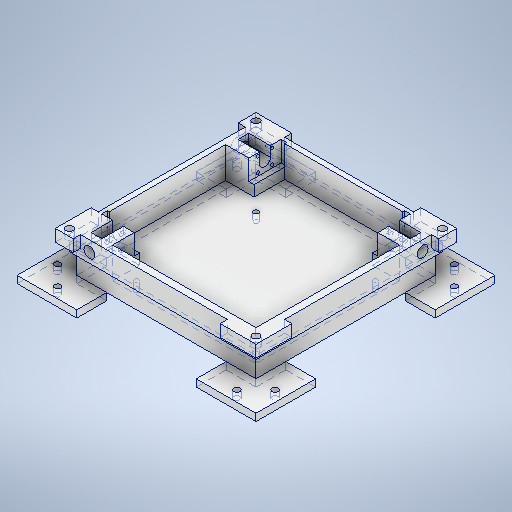
# Autodesk Inventor part: lower half
Saved by Autodesk Inventor 2025 (Build 290162000, 162)
## iProperties
Created: 2024-04-12
Part Number: lower half
Material: Aluminum 6061
Document SubType Name: Modeling
Designer: mahal
Density: 2.7 g/cm^3
Appearance: Aluminum - Flat
Mass: 892.67 g
Surface Area: 1106.39 cm^2
Volume: 330.618 cm^3
Author: mahal
Autodesk Inventor part; units mm, degrees
sketch "Sketch1" plane through (0, 0, 0) normal (0, 1, 0) x (-1, 0, 0)
  line L0 (75, 75) -> (-75, 75)
  line L1 (-75, 75) -> (-75, -75)
  line L2 (-75, -75) -> (75, -75)
  line L3 (75, -75) -> (75, 75)
  line L4 (75, 75) -> (-75, -75) construction
  line L5 (-75, 75) -> (75, -75) construction
  point P0 (0, 0)
  dimension "d0" = 150
  dimension "d1" = 150
  constraints: 12 end point, 2 midpoint, 2 parallel, 1 horizontal, 1 perpendicular
  measures "d0" distance of L2.end L1.end
  measures "d1" distance of L1.end L0.end
extrude "Extrusion1" add sketch "Sketch1" along normal blind 30
ref_plane "Work Plane1" through (0, 30, 0) normal (0, 1, 0) x (1, 0, 0)
sketch "Sketch2" plane through (0, 30, 0) normal (0, 1, 0) x (1, 0, 0)
  line L0 (72, -72) -> (-72, -72)
  line L1 (-72, -72) -> (-72, 72)
  line L2 (-72, 72) -> (72, 72)
  line L3 (72, 72) -> (72, -72)
  line L4 (72, -72) -> (-72, 72) construction
  line L5 (-72, -72) -> (72, 72) construction
  line L6 (72, -72) -> (-48, -72)
  line L7 (-48, -72) -> (-48, 48)
  line L8 (-48, 48) -> (72, 48)
  line L9 (72, 48) -> (72, -72)
  point P0 (0, 0)
  dimension "d5" = 144
  dimension "d6" = 144
  dimension "d7" = 120
  dimension "d8" = 120
  constraints: 20 end point, 4 parallel, 2 horizontal, 2 midpoint, 2 perpendicular
  measures "d5" distance of L1.end L2.end
  measures "d6" distance of L0.end L1.end
  measures "d7" distance of L7.end L8.end
  measures "d8" distance of L6.end L7.end
extrude "Extrusion2" cut sketch "Sketch2" against normal blind 26 contours L0 L7 L8 L3
sketch "Sketch3" plane through (0, 30, 0) normal (0, 1, 0) x (1, 0, 0)
  line L0 (72, -72) -> (-48, -72) projected
  line L1 (-48, -72) -> (-75, -72)
  line L2 (-75, 75) -> (-75, -75) projected
  line L3 (-61.5, -72) -> (-66, -72)
  line L4 (-61.5, -72) -> (-57, -72)
  line L5 (-57, -72) -> (-57, -54)
  line L6 (-57, -54) -> (-66, -54)
  line L7 (-66, -54) -> (-66, -72)
  line L8 (-57, -54) -> (-48, -54)
  line L9 (-48, -54) -> (-48, -49.5)
  line L10 (-48, -49.5) -> (-75, -49.5)
  line L11 (-75, -54) -> (-66, -54)
  line L12 (-75, -54) -> (-75, -49.5)
  line L13 (-48, 48) -> (72, 48) projected
  line L14 (72, 48) -> (72, 75)
  line L15 (72, 61.5) -> (72, 57)
  line L16 (72, 61.5) -> (72, 66)
  line L17 (72, 66) -> (54, 66)
  line L18 (54, 66) -> (54, 57)
  line L19 (54, 57) -> (72, 57)
  line L20 (54, 57) -> (54, 48)
  line L21 (54, 48) -> (49.5, 48)
  line L22 (49.5, 48) -> (49.5, 75)
  line L23 (75, 75) -> (-75, 75) projected
  line L24 (49.5, 75) -> (54, 75)
  line L25 (54, 75) -> (54, 66)
  line L26 (0, 48) -> (0, 57)
  line L27 (48, 48) -> (-72, 48)
  line L28 (-72, 48) -> (-72, 75)
  line L29 (-72, 61.5) -> (-72, 57)
  line L30 (-72, 61.5) -> (-72, 66)
  line L31 (-72, 66) -> (-54, 66)
  line L32 (-54, 66) -> (-54, 57)
  line L33 (-54, 57) -> (-72, 57)
  line L34 (-54, 57) -> (-54, 48)
  line L35 (-54, 48) -> (-49.5, 48)
  line L36 (-49.5, 48) -> (-49.5, 75)
  line L37 (-75, 75) -> (75, 75)
  line L38 (-49.5, 75) -> (-54, 75)
  line L39 (-54, 75) -> (-54, 66)
  point P0 (0, 0)
  dimension "d11" = 4.5
  dimension "d12" = 4.5
  dimension "d13" = 18
  dimension "d14" = 4.5
  dimension "d15" = 4.5
  dimension "d16" = 4.5
  dimension "d17" = 18
  dimension "d18" = 4.5
  constraints: 72 end point, 19 point on line, 14 symmetric about line, 12 perpendicular, 3 vertical, 2 horizontal, 2 midpoint, 1 collinear
  measures "d11" distance of L3.start L3.end
  measures "d12" distance of L3.start L4.end
  measures "d13" distance of L4.end L5.end
  measures "d14" distance of L8.end L9.end
  measures "d15" distance of L15.start L15.end
  measures "d16" distance of L15.start L16.end
  measures "d17" distance of L16.end L17.end
  measures "d18" distance of L20.end L21.end
extrude "Extrusion3" cut sketch "Sketch3" against normal blind 12.5 contours L1 L7 L6 L5 | L6 L11 L2 L10 L9 L8 | L23 L36 L27 L34 L32 L39 | L31 L32 L33 L28 | L23 L25 L18 L20 L13 L22 | L17 L14 L19 L18
sketch "Sketch5" plane through (0, 30, 0) normal (0, 1, 0) x (1, 0, 0)
  line L0 (54, 57) -> (54, 48) projected
  line L1 (49.5, 48) -> (49.5, 75) projected
  line L2 (54, 48) -> (49.5, 48)
  line L3 (49.5, 48) -> (49.5, 75)
  line L4 (49.5, 75) -> (54, 75)
  line L5 (54, 75) -> (54, 48)
  line L6 (-49.5, 75) -> (-49.5, 48) projected
  line L7 (-54, 66) -> (-54, 75) projected
  line L8 (-49.5, 48) -> (-54, 48)
  line L9 (-54, 48) -> (-54, 75)
  line L10 (-54, 75) -> (-49.5, 75)
  line L11 (-49.5, 75) -> (-49.5, 48)
  line L12 (-75, -49.5) -> (-48, -49.5) projected
  line L13 (-48, -54) -> (-75, -54)
  line L14 (-75, -54) -> (-75, -49.5)
  line L15 (-75, -49.5) -> (-48, -49.5)
  line L16 (-48, -49.5) -> (-48, -54)
  point P0 (0, 0)
  constraints: 24 end point, 6 parallel, 3 horizontal, 3 perpendicular
extrude "Extrusion4" cut sketch "Sketch5" against normal blind 17
sketch "Sketch6" plane through (0, 30, 0) normal (0, 1, 0) x (1, 0, 0)
  line L0 (49.5, 48) -> (49.5, 75) projected
  line L1 (49.5, 48) -> (-48.9491, 48)
  line L2 (-48.9491, 48) -> (-48.9491, 73.5)
  line L3 (-48.9491, 73.5) -> (49.5, 73.5)
  line L4 (49.5, 73.5) -> (49.5, 48)
  line L5 (-48, -49.5) -> (-48, 48) projected
  line L6 (-75, 75) -> (-75, -49.5) projected
  line L7 (-48, -49.5) -> (-75, -49.5)
  line L8 (-75, -49.5) -> (-75, 48)
  line L9 (-75, 48) -> (-48, 48)
  line L10 (-48, 48) -> (-48, -49.5)
  line L11 (-48, -49.5) -> (-73.5, -49.5)
  line L12 (-73.5, -49.5) -> (-73.5, 48)
  line L13 (-73.5, 48) -> (-48, 48)
  line L14 (-48, 48) -> (-48, -49.5)
  point P0 (0, 0)
  dimension "d23" = 25.5
  dimension "d24" = 25.5
  constraints: 24 end point, 6 parallel, 3 horizontal, 3 perpendicular, 3 point on line
  measures "d23" distance of L1.end L2.end
  measures "d24" distance of L12.end L13.end
extrude "Extrusion5" cut sketch "Sketch6" against normal up to surface (26 mm away) contours L1 L2 L3 L0 | L5 L7 L12 L9 L1
sketch "Sketch7" plane through (0, 30, 0) normal (0, 1, 0) x (1, 0, 0)
  line L0 (78, -78) -> (-78, -78)
  line L1 (-78, -78) -> (-78, 78)
  line L2 (-78, 78) -> (78, 78)
  line L3 (78, 78) -> (78, -78)
  line L4 (78, -78) -> (-78, 78) construction
  line L5 (-78, -78) -> (78, 78) construction
  line L6 (-75, 75) -> (-75, -49.5) projected
  line L7 (75, -75) -> (-75, -75)
  line L8 (-75, -75) -> (-75, 75)
  line L9 (-75, 75) -> (75, 75)
  line L10 (75, 75) -> (75, -75)
  line L11 (75, -75) -> (-75, 75) construction
  line L12 (-75, -75) -> (75, 75) construction
  point P0 (0, 0)
  dimension "d27" = 156
  dimension "d28" = 156
  constraints: 24 end point, 4 midpoint, 4 parallel, 2 horizontal, 2 perpendicular
  measures "d27" distance of L1.end L2.end
  measures "d28" distance of L0.end L1.end
extrude "Extrusion6" add sketch "Sketch7" against normal up to surface (17 mm away)
ref_plane "Work Plane2" through (-48.9491, 4, -73.5) normal (1, 0, 0) x (0, 0, -1)
sketch "Sketch8" plane through (-48.9491, 4, -73.5) normal (1, 0, 0) x (0, 0, -1)
  line L0 (-25.5, 26) -> (0, 26) projected
  line L1 (-25.5, 26) -> (0, 26)
  line L2 (0, 26) -> (0, 0)
  line L3 (0, 0) -> (-25.5, 0)
  line L4 (-25.5, 0) -> (-25.5, 26)
  point P0 (-73.5, -4)
  constraints: 8 end point, 2 parallel, 1 horizontal, 1 perpendicular
extrude "Extrusion7" cut sketch "Sketch8" against normal up to surface (0.5509 mm away)
sketch "Sketch9" plane through (0, 30, 0) normal (0, 1, 0) x (1, 0, 0)
  line L0 (-78, -78) -> (78, -78) projected
  line L1 (-78, -78) -> (-78, -54)
  line L2 (-78, 78) -> (-78, -78) projected
  line L3 (-78, -54) -> (-84, -54)
  line L4 (-84, -54) -> (-84, -78)
  line L5 (-84, -78) -> (-84, -84)
  line L6 (-84, -84) -> (-78, -84)
  line L7 (-78, -84) -> (-54, -84)
  line L8 (-54, -84) -> (-54, -78)
  line L9 (-78, -78) -> (-54, -78)
  line L10 (-78, 0) -> (-59.442, 0)
  line L11 (0, -78) -> (0, -66)
  line L12 (72, -72) -> (-48, -72) projected
  line L13 (-78, 78) -> (-78, 54)
  line L14 (-78, 54) -> (-84, 54)
  line L15 (-84, 54) -> (-84, 78)
  line L16 (-84, 78) -> (-84, 84)
  line L17 (-84, 84) -> (-78, 84)
  line L18 (-78, 84) -> (-54, 84)
  line L19 (-54, 84) -> (-54, 78)
  line L20 (-78, 78) -> (-54, 78)
  line L21 (78, -78) -> (-78, -78)
  line L22 (78, -78) -> (78, -54)
  line L23 (78, -54) -> (84, -54)
  line L24 (84, -54) -> (84, -78)
  line L25 (84, -78) -> (84, -84)
  line L26 (84, -84) -> (78, -84)
  line L27 (78, -84) -> (54, -84)
  line L28 (54, -84) -> (54, -78)
  line L29 (78, 78) -> (78, -78)
  line L30 (78, 78) -> (78, 54)
  line L31 (78, 54) -> (84, 54)
  line L32 (84, 54) -> (84, 78)
  line L33 (84, 78) -> (84, 84)
  line L34 (78, 84) -> (54, 84)
  line L35 (84, 84) -> (78, 84)
  line L36 (54, 84) -> (54, 78)
  line L37 (78, 78) -> (54, 78)
  point P0 (0, 0)
  dimension "d34" = 24
  dimension "d35" = 6
  dimension "d36" = 6
  dimension "d37" = 24
  constraints: 70 end point, 25 symmetric about line, 11 point on line, 4 perpendicular, 2 horizontal, 2 midpoint, 1 collinear
  measures "d34" distance of L0.start L1.end
  measures "d35" distance of L1.end L3.end
  measures "d36" distance of L4.end L5.end
  measures "d37" distance of L6.end L7.end
extrude "Extrusion8" add sketch "Sketch9" against normal blind 10
sketch "Sketch10" plane through (0, 30, 0) normal (0, 1, 0) x (1, 0, 0)
  line L0 (-84, 54) -> (-84, 84) projected
  line L1 (-78, 54) -> (-78, 78) projected
  line L2 (-84, 84) -> (-78, 84)
  line L3 (-78, 84) -> (-78, 78)
  line L4 (-78, 78) -> (-84, 78)
  line L5 (-84, 78) -> (-84, 84)
  circle A0 centre (-78, 78) radius 3
  line L6 (78, 78) -> (-78, 78) projected
  line L7 (0, 78) -> (0, 61.3441)
  line L8 (-78, 54) -> (-78, -54) projected
  line L9 (-78, 0) -> (-60.0355, 0)
  circle A1 centre (78, 78) radius 3
  circle A2 centre (-78, -78) radius 3
  circle A3 centre (78, -78) radius 3
  point P0 (0, 0)
  dimension "d40" = 6
  constraints: 12 end point, 4 centre point, 3 symmetric about line, 2 horizontal, 2 midpoint, 2 parallel, 1 coincident, 1 perpendicular, 1 vertical, 3 other
  measures "d40" diameter of A0
extrude "Extrusion9" cut sketch "Sketch10" against normal blind 7 contours A1 | A0 L3 L4 | L4 L1 A0 | L6 A0 L1 | L3 A0 L6 | A2 | A3
ref_plane "Work Plane3" through (0, 4, 0) normal (0, 1, 0) x (1, 0, 0)
sketch "Sketch11" plane through (0, 4, 0) normal (0, 1, 0) x (1, 0, 0)
  line L0 (72, -72) -> (-48, -72) projected
  line L1 (72, -72) -> (62, -72)
  line L2 (62, -72) -> (62, -62)
  line L3 (62, -62) -> (72, -62)
  line L4 (72, -62) -> (72, -72)
  circle A0 centre (62, -62) radius 2
  line L5 (72, -72) -> (-48, -72)
  line L6 (-48, -72) -> (-48, 48)
  line L7 (-48, 48) -> (72, 48)
  line L8 (72, 48) -> (72, -72)
  line L9 (12, -72) -> (12, -54.0613)
  line L10 (12, -12) -> (26.1191, -12)
  circle A1 centre (-38, -62) radius 2
  circle A2 centre (62, 38) radius 2
  circle A3 centre (-38, 38) radius 2
  point P0 (0, 0)
  dimension "d44" = 10
  dimension "d45" = 10
  dimension "d46" = 4
  dimension "d47" = 120
  dimension "d48" = 120
  constraints: 20 end point, 4 centre point, 4 parallel, 3 horizontal, 3 symmetric about line, 2 perpendicular, 1 coincident, 1 midpoint, 1 vertical, 3 other
  measures "d44" distance of L2.end L3.end
  measures "d45" distance of L1.end L2.end
  measures "d46" diameter of A0
  measures "d47" distance of L6.end L7.end
  measures "d48" distance of L5.end L6.end
extrude "Extrusion10" cut sketch "Sketch11" against normal blind 8 contours A0 L3 L2 | L2 L3 A0 | A1 | A2 | A3
ref_plane "Work Plane4" through (0, 0, 0) normal (0, -1, 0) x (1, 0, 0)
sketch "Sketch12" plane through (0, 0, 0) normal (0, -1, 0) x (1, 0, 0)
  line L0 (-75, 75) -> (75, 75) projected
  line L1 (-75, 75) -> (75, 75)
  line L2 (75, 75) -> (75, -75)
  line L3 (75, -75) -> (-75, -75)
  line L4 (-75, -75) -> (-75, 75)
  point P0 (0, 0)
  constraints: 8 end point, 2 parallel, 1 horizontal, 1 perpendicular
extrude "Extrusion11" add sketch "Sketch12" along normal blind 4
ref_plane "Work Plane5" through (0, -4, 0) normal (0, -1, 0) x (1, 0, 0)
sketch "Sketch13" plane through (0, -4, 0) normal (0, -1, 0) x (1, 0, 0)
  line L0 (-100, -100) -> (100, -100)
  line L1 (100, -100) -> (100, 100)
  line L2 (100, 100) -> (-100, 100)
  line L3 (-100, 100) -> (-100, -100)
  line L4 (-100, -100) -> (100, 100) construction
  line L5 (100, -100) -> (-100, 100) construction
  line L6 (75, -75) -> (75, 75) projected
  line L7 (-75, -75) -> (75, -75)
  line L8 (75, -75) -> (75, 75)
  line L9 (75, 75) -> (-75, 75)
  line L10 (-75, 75) -> (-75, -75)
  line L11 (-75, -75) -> (75, 75) construction
  line L12 (75, -75) -> (-75, 75) construction
  line L13 (-100, -100) -> (-50, -100)
  line L14 (-50, -100) -> (-50, -50)
  line L15 (-50, -50) -> (-100, -50)
  line L16 (-100, -50) -> (-100, -100)
  line L17 (-100, -100) -> (-50, -50) construction
  line L18 (-50, -100) -> (-100, -50) construction
  line L19 (-100, 50) -> (-50, 50)
  line L20 (-50, 50) -> (-50, 100)
  line L21 (-50, 100) -> (-100, 100)
  line L22 (-100, 100) -> (-100, 50)
  line L23 (-100, 50) -> (-50, 100) construction
  line L24 (-50, 50) -> (-100, 100) construction
  line L25 (50, 50) -> (100, 50)
  line L26 (100, 50) -> (100, 100)
  line L27 (100, 100) -> (50, 100)
  line L28 (50, 100) -> (50, 50)
  line L29 (50, 50) -> (100, 100) construction
  line L30 (100, 50) -> (50, 100) construction
  line L31 (50, -100) -> (100, -100)
  line L32 (100, -100) -> (100, -50)
  line L33 (100, -50) -> (50, -50)
  line L34 (50, -50) -> (50, -100)
  line L35 (50, -100) -> (100, -50) construction
  line L36 (100, -100) -> (50, -50) construction
  point P0 (0, 0)
  point P1 (50, -75)
  point P2 (75, -50)
  point P3 (50, 75)
  point P4 (75, 50)
  point P5 (-50, 75)
  point P6 (-75, 50)
  point P7 (-75, -50)
  point P8 (-50, -75)
  dimension "d55" = 200
  dimension "d56" = 200
  dimension "d57" = 50
  dimension "d58" = 50
  dimension "d59" = 50
  dimension "d60" = 50
  dimension "d61" = 50
  dimension "d62" = 50
  dimension "d63" = 50
  constraints: 72 end point, 12 midpoint, 12 parallel, 6 horizontal, 6 perpendicular, 1 point on line
  measures "d55" distance of L2.end L1.end
  measures "d56" distance of L1.end L0.end
  measures "d57" distance of L15.end L14.end
  measures "d58" distance of L21.end L20.end
  measures "d59" distance of L20.end L19.end
  measures "d60" distance of L27.end L1.end
  measures "d61" distance of L1.end L25.end
  measures "d62" distance of L33.end L32.end
  measures "d63" distance of L32.end L31.end
extrude "Extrusion12" add sketch "Sketch13" along normal blind 6 contours L3 L15 L10 L7 L14 L0 | L34 L7 L6 L33 L1 L0 | L3 L2 L20 L9 L10 L19 | L25 L6 L9 L28 L2 L1
ref_plane "Work Plane6" through (0, -4, 0) normal (0, 1, 0) x (1, 0, 0)
sketch "Sketch14" plane through (0, -4, 0) normal (0, 1, 0) x (1, 0, 0)
  line L0 (100, -50) -> (100, -100) projected
  line L1 (100, -100) -> (100, -50)
  line L2 (50, -100) -> (50, -75) projected
  line L3 (100, -100) -> (50, -100)
  line L4 (75, -100) -> (75, -91)
  line L5 (100, -75) -> (91, -75)
  circle A0 centre (91, -75) radius 2.5
  circle A1 centre (75, -91) radius 2.5
  line L6 (-78, -78) -> (78, -78) projected
  line L7 (0, -78) -> (0, -91)
  line L8 (78, 0) -> (95.5, 0)
  circle A2 centre (-91, -75) radius 2.5
  circle A3 centre (-75, -91) radius 2.5
  circle A4 centre (91, 75) radius 2.5
  circle A5 centre (75, 91) radius 2.5
  circle A6 centre (-75, 91) radius 2.5
  circle A7 centre (-91, 75) radius 2.5
  point P0 (0, 0)
  dimension "d67" = 9
  dimension "d68" = 9
  dimension "d69" = 5
  dimension "d70" = 5
  constraints: 12 end point, 8 centre point, 6 symmetric about line, 3 midpoint, 2 coincident, 2 horizontal, 2 vertical, 1 collinear, 1 perpendicular, 6 other
  measures "d67" distance of L4.start L4.end
  measures "d68" distance of L5.start L5.end
  measures "d69" diameter of A0
  measures "d70" diameter of A1
extrude "Extrusion13" cut sketch "Sketch14" against normal up to surface (6 mm away)
ref_plane "Work Plane7" through (72, 17.5, -66) normal (-1, 0, 0) x (0, 0, 1)
sketch "Sketch15" plane through (72, 17.5, -66) normal (-1, 0, 0) x (0, 0, 1)
  line L0 (0, 12.5) -> (9, 12.5) projected
  line L1 (4.5, 12.5) -> (4.5, 4)
  circle A0 centre (4.5, 4) radius 4.5
  point P0 (66, -17.5)
  dimension "d74" = 8.5
  dimension "d75" = 9
  constraints: 2 end point, 1 centre point, 1 coincident, 1 midpoint, 1 vertical
  measures "d74" distance of L1.start L1.end
  measures "d75" diameter of A0
extrude "Extrusion14" cut sketch "Sketch15" against normal up to surface (12 mm away)
ref_plane "Work Plane8" through (-72, 17.5, -57) normal (1, 0, 0) x (0, 0, -1)
sketch "Sketch16" plane through (-72, 17.5, -57) normal (1, 0, 0) x (0, 0, -1)
  line L0 (0, 12.5) -> (9, 12.5) projected
  line L1 (4.5, 12.5) -> (4.5, 4)
  circle A0 centre (4.5, 4) radius 4.5
  point P0 (-57, -17.5)
  dimension "d79" = 8.5
  dimension "d80" = 9
  constraints: 2 end point, 1 centre point, 1 coincident, 1 midpoint, 1 vertical
  measures "d79" distance of L1.start L1.end
  measures "d80" diameter of A0
extrude "Extrusion15" cut sketch "Sketch16" against normal up to surface (12 mm away)
ref_plane "Work Plane9" through (-57, 30, 72) normal (0, 0, -1) x (-1, 0, 0)
sketch "Sketch17" plane through (-57, 30, 72) normal (0, 0, -1) x (-1, 0, 0)
  line L0 (0, 0) -> (9, 0) projected
  line L1 (4.5, 0) -> (4.5, -9)
  circle A0 centre (4.5, -9) radius 4.5
  point P0 (-57, -30)
  dimension "d84" = 9
  dimension "d85" = 9
  constraints: 2 end point, 1 centre point, 1 coincident, 1 midpoint, 1 vertical
  measures "d84" distance of L1.start L1.end
  measures "d85" diameter of A0
extrude "Extrusion16" cut sketch "Sketch17" against normal up to surface (12 mm away)
ref_plane "Work Plane10" through (0, 30, 0) normal (0, 1, 0) x (1, 0, 0)
sketch "Sketch18" plane through (0, 30, 0) normal (0, 1, 0) x (1, 0, 0)
  line L0 (78, -54) -> (78, 54) projected
  line L1 (84, 54) -> (84, 84) projected
  line L2 (78, 54) -> (84, 54)
  line L3 (84, 54) -> (84, 69)
  line L4 (84, 69) -> (78, 69)
  line L5 (78, 69) -> (78, 54)
  line L6 (-84, 84) -> (-84, 54) projected
  line L7 (-78, 54) -> (-84, 54)
  line L8 (-84, 54) -> (-84, 69)
  line L9 (-84, 69) -> (-78, 69)
  line L10 (-78, 69) -> (-78, 54)
  line L11 (-54, -78) -> (-54, -84) projected
  line L12 (-65.8875, -84) -> (-84, -84) projected
  line L13 (-54, -78) -> (-69, -78)
  line L14 (-69, -78) -> (-69, -84)
  line L15 (-69, -84) -> (-54, -84)
  line L16 (-54, -84) -> (-54, -78)
  point P0 (0, 0)
  dimension "d89" = 15
  constraints: 24 end point, 6 parallel, 3 horizontal, 3 perpendicular, 2 midpoint, 2 point on line
  measures "d89" distance of L15.end L14.end
extrude "Extrusion17" cut sketch "Sketch18" against normal up to surface (10 mm away)
sketch "Sketch19" plane through (72, 17.5, -66) normal (-1, 0, 0) x (0, 0, 1)
  arc A0 (9, 4) -> (0, 4) centre (4.5, 4) ccw projected
  circle A1 centre (4.5, 4) radius 4.5
  line L0 (0, 4) -> (9, 4)
  line L1 (9, 4) -> (9, -0.5)
  line L2 (9, -0.5) -> (0, -0.5)
  line L3 (0, -0.5) -> (0, 4)
  point P0 (66, -17.5)
  point P1 (4.5, -0.5)
  constraints: 8 end point, 2 parallel, 1 centre point, 1 coincident, 1 horizontal, 1 perpendicular
extrude "Extrusion18" add sketch "Sketch19" along normal up to surface (18 mm away) contours L1 L2 A1 | A1 L2 L3
sketch "Sketch20" plane through (72, 17.5, -66) normal (-1, 0, 0) x (0, 0, 1)
  arc A0 (9, 4) -> (0, 4) centre (4.5, 4) ccw projected
  circle A1 centre (4.5, 4) radius 4.5
  point P0 (66, -17.5)
  constraints: 1 centre point, 1 coincident
extrude "Extrusion19" cut sketch "Sketch20" along normal up to surface (18 mm away)
sketch "Sketch21" plane through (-72, 17.5, -57) normal (1, 0, 0) x (0, 0, -1)
  arc A0 (9, 4) -> (0, 4) centre (4.5, 4) ccw projected
  circle A1 centre (4.5, 4) radius 4.5
  line L0 (0, 4) -> (9, 4)
  line L1 (9, 4) -> (9, -0.5)
  line L2 (9, -0.5) -> (0, -0.5)
  line L3 (0, -0.5) -> (0, 4)
  point P0 (-57, -17.5)
  point P1 (4.5, -0.5)
  constraints: 8 end point, 2 parallel, 1 centre point, 1 coincident, 1 horizontal, 1 perpendicular
extrude "Extrusion20" add sketch "Sketch21" along normal up to surface (18 mm away) contours L1 L2 A1 | A1 L2 L3
sketch "Sketch22" plane through (-72, 17.5, -57) normal (1, 0, 0) x (0, 0, -1)
  arc A0 (9, 4) -> (0, 4) centre (4.5, 4) ccw projected
  circle A1 centre (4.5, 4) radius 4.5
  point P0 (-57, -17.5)
  constraints: 1 centre point, 1 coincident
extrude "Extrusion21" cut sketch "Sketch22" along normal up to surface (18 mm away)
sketch "Sketch23" plane through (-57, 30, 72) normal (0, 0, -1) x (-1, 0, 0)
  arc A0 (9, -9) -> (0, -9) centre (4.5, -9) ccw projected
  circle A1 centre (4.5, -9) radius 4.5
  line L0 (9, -9) -> (0, -9)
  line L1 (0, -9) -> (0, -13.5)
  line L2 (0, -13.5) -> (9, -13.5)
  line L3 (9, -13.5) -> (9, -9)
  point P0 (-57, -30)
  point P1 (4.5, -13.5)
  constraints: 8 end point, 2 parallel, 1 centre point, 1 coincident, 1 horizontal, 1 perpendicular
extrude "Extrusion22" add sketch "Sketch23" along normal up to surface (18 mm away) contours L3 L2 A1 | A1 L2 L1
sketch "Sketch24" plane through (-57, 30, 72) normal (0, 0, -1) x (-1, 0, 0)
  arc A0 (9, -9) -> (0, -9) centre (4.5, -9) ccw projected
  circle A1 centre (4.5, -9) radius 4.5
  point P0 (-57, -30)
  constraints: 1 centre point, 1 coincident
extrude "Extrusion23" cut sketch "Sketch24" along normal up to surface (18 mm away)
ref_plane "Work Plane11" through (54, 30, -57) normal (-1, 0, 0) x (0, 0, 1)
sketch "Sketch25" plane through (54, 30, -57) normal (-1, 0, 0) x (0, 0, 1)
  line L0 (-18, -17) -> (-18, 0) projected
  line L1 (-18, 0) -> (9, 0)
  line L2 (9, 0) -> (9, -17)
  line L3 (9, -17) -> (-18, -17)
  line L4 (-18, -17) -> (-18, 0)
  line L5 (-13, 0) -> (4, 0)
  line L6 (4, 0) -> (4, -17)
  line L7 (4, -17) -> (-13, -17)
  line L8 (-13, -17) -> (-13, 0)
  arc A0 (-9, -8.5) -> (0, -8.5) centre (-4.5, -8.5) ccw projected
  line L9 (-13, 0) -> (4, -17) construction
  line L10 (4, 0) -> (-13, -17) construction
  line L11 (-10.5, -2.5) -> (1.5, -2.5)
  line L12 (1.5, -2.5) -> (1.5, -14.5)
  line L13 (1.5, -14.5) -> (-10.5, -14.5)
  line L14 (-10.5, -14.5) -> (-10.5, -2.5)
  line L15 (-10.5, -2.5) -> (1.5, -14.5) construction
  line L16 (1.5, -2.5) -> (-10.5, -14.5) construction
  circle A1 centre (-10.5, -2.5) radius 1.25
  circle A2 centre (1.5, -2.5) radius 1.25
  circle A3 centre (1.5, -14.5) radius 1.25
  circle A4 centre (-10.5, -14.5) radius 1.25
  point P0 (57, -30)
  dimension "d105" = 17
  dimension "d106" = 12
  dimension "d107" = 12
  dimension "d108" = 2.5
  dimension "d109" = 2.5
  dimension "d110" = 2.5
  dimension "d111" = 2.5
  constraints: 32 end point, 6 parallel, 4 centre point, 4 coincident, 4 midpoint, 3 horizontal, 3 perpendicular, 1 point on line
  measures "d105" distance of L6.end L7.end
  measures "d106" distance of L12.end L13.end
  measures "d107" distance of L11.end L12.end
  measures "d108" diameter of A1
  measures "d109" diameter of A2
  measures "d110" diameter of A3
  measures "d111" diameter of A4
extrude "Extrusion24" cut sketch "Sketch25" against normal blind 4 contours L14 A1 L11 | L11 A1 L14 | A2 L12 L11 | L11 L12 A2 | A4 L13 L14 | L14 L13 A4 | A3 L13 L12 | L12 L13 A3
ref_plane "Work Plane12" through (-54, 13, -48) normal (1, 0, 0) x (0, 0, -1)
sketch "Sketch26" plane through (-54, 13, -48) normal (1, 0, 0) x (0, 0, -1)
  line L0 (5, 17) -> (22, 17)
  line L1 (22, 17) -> (22, 0)
  line L2 (22, 0) -> (5, 0)
  line L3 (5, 0) -> (5, 17)
  arc A0 (9, 8.5) -> (18, 8.5) centre (13.5, 8.5) ccw projected
  line L4 (5, 17) -> (22, 0) construction
  line L5 (22, 17) -> (5, 0) construction
  line L6 (7.5, 14.5) -> (19.5, 14.5)
  line L7 (19.5, 14.5) -> (19.5, 2.5)
  line L8 (19.5, 2.5) -> (7.5, 2.5)
  line L9 (7.5, 2.5) -> (7.5, 14.5)
  line L10 (7.5, 14.5) -> (19.5, 2.5) construction
  line L11 (19.5, 14.5) -> (7.5, 2.5) construction
  circle A1 centre (7.5, 14.5) radius 1.25
  circle A2 centre (19.5, 14.5) radius 1.25
  circle A3 centre (19.5, 2.5) radius 1.25
  circle A4 centre (7.5, 2.5) radius 1.25
  point P0 (-48, -13)
  dimension "d115" = 17
  dimension "d116" = 17
  dimension "d117" = 12
  dimension "d118" = 12
  dimension "d119" = 2.5
  dimension "d120" = 2.5
  dimension "d121" = 2.5
  dimension "d122" = 2.5
  constraints: 24 end point, 5 midpoint, 4 centre point, 4 coincident, 4 parallel, 2 horizontal, 2 perpendicular
  measures "d115" distance of L1.end L2.end
  measures "d116" distance of L0.end L1.end
  measures "d117" distance of L7.end L8.end
  measures "d118" distance of L6.end L7.end
  measures "d119" diameter of A1
  measures "d120" diameter of A2
  measures "d121" diameter of A3
  measures "d122" diameter of A4
extrude "Extrusion25" cut sketch "Sketch26" against normal blind 4 contours L9 A1 L6 | L6 A1 L9 | A2 L7 L6 | L6 L7 A2 | A4 L8 L9 | L9 L8 A4 | A3 L8 L7 | L7 L8 A3
ref_plane "Work Plane13" through (-48, 30, 54) normal (0, 0, -1) x (-1, 0, 0)
sketch "Sketch27" plane through (-48, 30, 54) normal (0, 0, -1) x (-1, 0, 0)
  line L0 (5, -0.5) -> (22, -0.5)
  line L1 (22, -0.5) -> (22, -17.5)
  line L2 (22, -17.5) -> (5, -17.5)
  line L3 (5, -17.5) -> (5, -0.5)
  arc A0 (9, -9) -> (18, -9) centre (13.5, -9) ccw projected
  line L4 (5, -0.5) -> (22, -17.5) construction
  line L5 (22, -0.5) -> (5, -17.5) construction
  line L6 (7.5, -3) -> (19.5, -3)
  line L7 (19.5, -3) -> (19.5, -15)
  line L8 (19.5, -15) -> (7.5, -15)
  line L9 (7.5, -15) -> (7.5, -3)
  arc A1 (9.1125, -10) -> (17.8875, -10) centre (13.5, -9) ccw projected
  line L10 (7.5, -3) -> (19.5, -15) construction
  line L11 (19.5, -3) -> (7.5, -15) construction
  circle A2 centre (7.5, -3) radius 1.25
  circle A3 centre (19.5, -3) radius 1.25
  circle A4 centre (7.5, -15) radius 1.25
  circle A5 centre (19.5, -15) radius 1.25
  point P0 (-48, -30)
  dimension "d126" = 17
  dimension "d127" = 17
  dimension "d128" = 12
  dimension "d129" = 12
  dimension "d130" = 2.5
  dimension "d131" = 2.5
  dimension "d132" = 2.5
  dimension "d133" = 2.5
  constraints: 24 end point, 4 centre point, 4 coincident, 4 midpoint, 4 parallel, 2 horizontal, 2 perpendicular
  measures "d126" distance of L1.end L2.end
  measures "d127" distance of L0.end L1.end
  measures "d128" distance of L7.end L8.end
  measures "d129" distance of L6.end L7.end
  measures "d130" diameter of A2
  measures "d131" diameter of A3
  measures "d132" diameter of A4
  measures "d133" diameter of A5
extrude "Extrusion26" cut sketch "Sketch27" against normal blind 4 contours L9 A2 L6 | L6 A2 L9 | A3 L7 L6 | L6 L7 A3 | A4 L8 L9 | L9 L8 A4 | A5 L8 L7 | L7 L8 A5
thread "Thread1" size "M2x0.4" class "6H" standard "ANSI Metric M Profile" full length
thread "Thread2" size "M2x0.4" class "6H" standard "ANSI Metric M Profile" full length
thread "Thread3" size "M2x0.4" class "6H" standard "ANSI Metric M Profile" full length
thread "Thread4" size "M2x0.4" class "6H" standard "ANSI Metric M Profile" full length
thread "Thread5" size "M2x0.4" class "6H" standard "ANSI Metric M Profile" full length
thread "Thread6" size "M2x0.4" class "6H" standard "ANSI Metric M Profile" full length
thread "Thread7" size "M2x0.4" class "6H" standard "ANSI Metric M Profile" full length
thread "Thread8" size "M2x0.4" class "6H" standard "ANSI Metric M Profile" full length
thread "Thread9" size "M2x0.4" class "6H" standard "ANSI Metric M Profile" full length
thread "Thread10" size "M2x0.4" class "6H" standard "ANSI Metric M Profile" full length
thread "Thread11" size "M2x0.4" class "6H" standard "ANSI Metric M Profile" full length
thread "Thread12" size "M2x0.4" class "6H" standard "ANSI Metric M Profile" full length
ref_plane "Work Plane14" through (62, 0, -38) normal (0, 1, 0) x (1, 0, 0)
sketch "Sketch28" plane through (62, 0, -38) normal (0, 1, 0) x (1, 0, 0)
  circle A0 centre (0, 0) radius 2
  circle A1 centre (0, -100) radius 2 projected
  circle A2 centre (0, -100) radius 4.5
  circle A3 centre (-100, -100) radius 2 projected
  circle A4 centre (-100, -100) radius 4.5
  circle A5 centre (-100, 0) radius 2 projected
  circle A6 centre (-100, 0) radius 4.5
  point P0 (-62, -38)
  dimension "d163" = 4
  constraints: 4 centre point, 3 coincident
  measures "d163" diameter of A0
extrude "Extrusion27" cut sketch "Sketch28" against normal blind 3 contours A0 | A1 | A3 | A5
body "Solid1"
